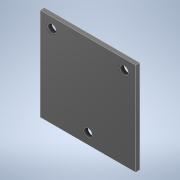
# Autodesk Inventor part: PCB-EncoderMain
Saved by Autodesk Inventor 2022 (Build 260153000, 153)
## iProperties
Created: 2024-07-02
Part Number: PCB-EncoderMain
Material: 一般
Document SubType Name: Modeling
Designer: yamashita1
Density: 1 g/cm^3
Appearance: 滑らか - 黒
Author: yamashita1
Autodesk Inventor part; units mm, degrees
ref_plane "YZ Plane" through (0, 0, 0) normal (1, 0, 0) x (0, 1, 0)
ref_plane "XZ Plane" through (0, 0, 0) normal (0, 1, 0) x (-1, 0, 0)
ref_plane "XY Plane" through (0, 0, 0) normal (0, 0, 1) x (1, 0, 0)
sketch "スケッチ1" plane through (0, 0, 0) normal (0, 0, 1) x (1, 0, 0)
  line L0 (-18.5, 36) -> (18.5, 36)
  line L1 (18.5, 36) -> (18.5, 0)
  line L2 (18.5, 0) -> (-18.5, 0)
  line L3 (-18.5, 0) -> (-18.5, 36)
  circle A0 centre (0, 4) radius 1.6
  circle A1 centre (14, 32) radius 1.6
  circle A2 centre (-14, 32) radius 1.6
  line L4 (0, 42.25) -> (0, -4.7356) construction
  point P0 (0, 0)
  point P1 (0, 0)
  dimension "d0" = 37
  dimension "d1" = 36
  dimension "d2" = 3.2
  dimension "d3" = 4
  dimension "d4" = 4
  dimension "d5" = 4.5
  constraints: 10 end point, 3 centre point, 2 equal radius, 2 parallel, 2 point on line, 1 coincident, 1 horizontal, 1 horizontal alignment, 1 midpoint, 1 perpendicular, 1 symmetric about line, 1 vertical
  measures "d0" distance of L1.end L2.end
  measures "d1" distance of L0.end L1.end
  measures "d2" diameter of A0
  measures "d3" distance from line of L2 A0.centre
  measures "d4" distance from line of L0 A1.centre
  measures "d5" distance from line of L1 A1.centre
extrude "押し出し1" add sketch "スケッチ1" along normal blind 1.6
